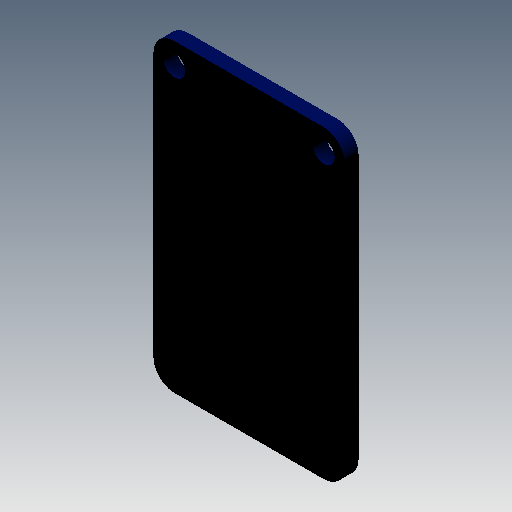
# Autodesk Inventor part: PowerBoost500
Saved by Autodesk Inventor 2017 (Build 210142000, 142)
## iProperties
GlobalPropertyList: <PropertyList/>
Part Number: PowerBoost500
Material: Generisch
Document SubType Name: Modeling
Designer: Werkstatt
Density: 1 g/cm^3
Appearance: Vorgabe(1)
Author: Werkstatt
Autodesk Inventor part; units mm, degrees
ref_plane "YZ Plane" through (0, 0, 0) normal (1, 0, 0) x (0, 1, 0)
ref_plane "XZ Plane" through (0, 0, 0) normal (0, 1, 0) x (-1, 0, 0)
ref_plane "XY Plane" through (0, 0, 0) normal (0, 0, 1) x (1, 0, 0)
sketch "Skizze1" plane through (0, 0, 0) normal (0, 1, 0) x (-1, 0, 0)
  line L0 (-11.455, -18.25) -> (11.455, -18.25)
  line L1 (11.455, -18.25) -> (11.455, 18.25)
  line L2 (11.455, 18.25) -> (-11.455, 18.25)
  line L3 (-11.455, 18.25) -> (-11.455, -18.25)
  line L4 (-11.455, -18.25) -> (11.455, 18.25) construction
  line L5 (11.455, -18.25) -> (-11.455, 18.25) construction
  point P0 (0, 0)
  dimension "d0" = 22.91
  dimension "d1" = 36.5
  constraints: 12 end point, 2 midpoint, 2 parallel, 1 horizontal, 1 perpendicular
  measures "d0" distance of L2.end L1.end
  measures "d1" distance of L1.end L0.end
extrude "Extrusion1" add sketch "Skizze1" along normal blind 1.67
fillet "Rundung1" radius 2.5 4 edges at (-11.455, 0.835, 18.25) (11.455, 0.835, -18.25) (11.455, 0.835, 18.25) (-11.455, 0.835, -18.25)
sketch "Skizze2" plane through (0, 1.67, 0) normal (0, 1, 0) x (1, 0, 0)
  circle A0 centre (-8.955, -15.75) radius 1.3
  line L0 (-8.955, -18.25) -> (8.955, -18.25) projected
  line L1 (-11.455, 15.75) -> (-11.455, -15.75) projected
  line L2 (0, 0) -> (0, -21.9467) construction
  circle A1 centre (8.955, -15.75) radius 1.3
  dimension "d5" = 2.6
  dimension "d6" = 2.5
  dimension "d7" = 2.5
  dimension "d8" = 17.91
  constraints: 2 centre point, 2 end point, 1 symmetric about line, 1 vertical, 1 other
  measures "d5" diameter of A0
  measures "d6" distance from line of L0 A0.centre
  measures "d7" distance from line of L1 A0.centre
  measures "d8" distance of A1.centre A0.centre
extrude "Extrusion2" cut sketch "Skizze2" against normal up to next
